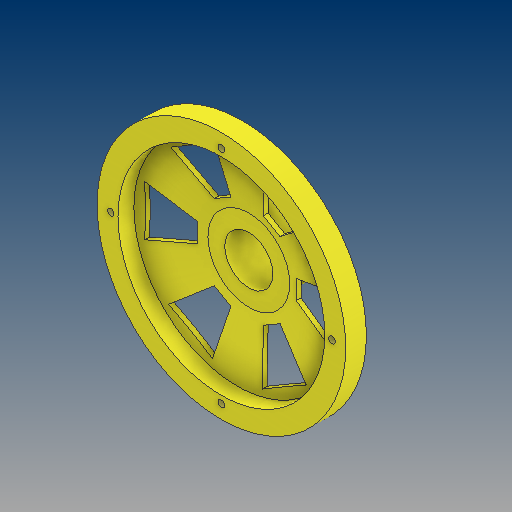
# Autodesk Inventor part: ring_1-sun_2
Saved by Autodesk Inventor 2021 (Build 250183000, 183)
## iProperties
Created: 2020-12-25
Part Number: ring_1-sun_2
Material: Generic
Document SubType Name: Modeling
Designer: Διογενης Τσιχλακης
Density: 1 g/cm^3
Appearance: Default
Mass: 1678.65 g
Surface Area: 4498.74 cm^2
Volume: 1678.65 cm^3
Sending System: Autodesk Inventor 2021
Preprocessor: unknown
Minimum Resolution: 0.01
Sent Units: Millimeter
Translation Standard: IGES 5.3
Model Creation Time: 2020-12-25
Title: sun_2_narrow
Author: Angelos
Autodesk Inventor part; units mm, degrees
ref_plane "YZ Plane" through (0, 0, 0) normal (1, 0, 0) x (0, 1, 0)
ref_plane "XZ Plane" through (0, 0, 0) normal (0, 1, 0) x (-1, 0, 0)
ref_plane "Work Plane1" through (-79.7284, -22.4294, -13.998) normal (0, 0, -1) x (-0.9355686, -0.3531449, 0)
sketch "Sketch5" plane through (-79.7284, -22.4294, -13.998) normal (0, 0, -1) x (-0.9355686, -0.3531449, 0)
  circle A0 centre (-82.5122, -7.1715) radius 70
  circle A1 centre (-82.5122, -7.1715) radius 50
  dimension "d4" = 100
  dimension "d30" = 140
  constraints: 2 centre point, 2 coincident
  measures "d4" diameter of A1
  measures "d30" diameter of A0
extrude "Extrusion2" add sketch "Sketch5" against normal blind 77
sketch "Sketch6" plane through (0, 0, 63.002) normal (0, 0, 1) x (1, 0, 0)
  circle A0 centre (0, 0) radius 85
  circle A1 centre (0, 0) radius 50
  dimension "d7" = 170
  dimension "d8" = 100
  constraints: 2 centre point, 2 coincident
  measures "d7" diameter of A0
  measures "d8" diameter of A1
extrude "Extrusion3" add sketch "Sketch6" along normal blind 10
sketch "Sketch7" plane through (0, 0, 0) normal (0, 1, 0) x (-1, 0, 0)
  line L0 (85, 73.002) -> (-85, 73.002) projected
  line L1 (-215, 97) -> (-85, 73.002)
  line L2 (85, 63.002) -> (-85, 63.002) projected
  line L3 (-85, 73.002) -> (-85, 63.002)
  line L4 (-215, 97) -> (-215, 87)
  line L5 (-215, 87) -> (-85, 63.002)
  line L6 (-230, 87) -> (-215, 87)
  line L7 (-215, 97) -> (-230, 97)
  line L8 (0, -19.4) -> (0, 116.4) projected
  line L9 (-258.5, 87) -> (-258.5, 97)
  line L10 (-258.5, 97) -> (-230, 97)
  line L11 (0, 62) -> (-85, 62)
  line L12 (-215, 87) -> (-258.5, 87)
  point P0 (0, 0)
  dimension "d32" = 10
  dimension "d59" = 258.5
  constraints: 20 end point, 4 perpendicular, 3 horizontal, 2 point on line, 1 vertical
  measures "d32" distance between parallel lines of L6 L7
  measures "d59" distance from line of L8 L9.end
revolve "Revolution1" add sketch "Sketch7" angle 360 about axis through (0, 0, -10) along (0, 0, 1) contours L3 L5 L4 L1 | L4 L6 L12 L9 L10 L7
sketch "Sketch9" plane through (0, 0, 0) normal (0, 0, 1) x (1, 0, 0)
  line L0 (194.9339, 0) -> (194.9339, -55)
  line L1 (194.9339, 0) -> (194.9339, 50)
  line L2 (102.2316, 0) -> (102.2316, 20)
  line L3 (102.2316, 0) -> (102.2316, -20)
  line L4 (102.2316, -20) -> (194.9339, -55)
  line L5 (102.2316, 20) -> (194.9339, 50)
  point P0 (0, 0)
  constraints: 12 end point, 4 vertical
extrude "Extrusion5" cut sketch "Sketch9" along normal through all
pattern_circular "Circular Pattern2" count 6 over 360 about axis through (0, 0, -10) along (0, 0, 1) of "Extrusion5"
sketch "Sketch11" plane through (0, 0, 97) normal (0, 0, 1) x (1, 0, 0)
  circle A0 centre (0, 0) radius 258.5
  circle A1 centre (0, 0) radius 215
  dimension "d58" = 517
  constraints: 2 centre point, 2 coincident
  measures "d58" diameter of A0
extrude "Extrusion9" add sketch "Sketch11" along normal blind 33.07
sketch "Sketch12" plane through (0, 0, 130.07) normal (0, 0, 1) x (1, 0, 0)
  circle A0 centre (0, 230) radius 7
  point P0 (0, 0)
  dimension "d41" = 14
  dimension "d42" = 230
  constraints: 1 centre point
  measures "d41" diameter of A0
  measures "d42" distance of A0.centre point (0, 0)
extrude "Extrusion10" cut sketch "Sketch12" against normal blind 25
pattern_circular "Circular Pattern4" count 4 over 360 about axis through (0, 0, -13.998) along (0, 0, 1) of "Extrusion10"
sketch "Sketch14" plane through (0, 0, 0) normal (1, 0, 0) x (0, 1, 0)
  line L0 (237, 105.07) -> (227, 105.07)
  line L1 (230, 119.807) -> (237, 123.07)
  line L2 (237, 123.07) -> (230, 123.07)
  line L3 (223, 105.07) -> (237, 105.07) projected
  line L4 (230, 123.07) -> (230, 119.807)
  point P0 (0, 0)
  constraints: 8 end point, 1 horizontal, 1 perpendicular, 1 other
thread "Thread5" size "M14x2" class "6H" standard "ANSI Metric M Profile" full length
thread "Thread6" size "M14x2" class "6H" standard "ANSI Metric M Profile" full length
thread "Thread7" size "M14x2" class "6H" standard "ANSI Metric M Profile" full length
thread "Thread8" size "M14x2" class "6H" standard "ANSI Metric M Profile" full length
revolve "Revolution4" cut sketch "Sketch14" angle 360 about axis through (0, 230, 123.07) along (0, 0, -1)
pattern_circular "Circular Pattern5" count 4 over 360 about axis through (0, 0, 97) along (0, 0, 1) of "Revolution4"
sketch "Sketch16" plane through (0, 0, -13.998) normal (0, 0, -1) x (-1, 0, 0)
  circle A0 centre (-59, 0) radius 6
  circle A1 centre (0, 0) radius 85 projected
  dimension "d77" = 59
  dimension "d78" = 12
  constraints: 1 centre point
  measures "d77" distance of A1.centre A0.centre
  measures "d78" diameter of A0
extrude "Extrusion12" cut sketch "Sketch16" against normal blind 10 contours A0
sketch "Sketch17" plane through (0, 0, 0) normal (0, 1, 0) x (-1, 0, 0)
  line L0 (-53, -3.998) -> (-65, -3.998) projected
  line L1 (-70, -13.998) -> (70, -13.998) projected
  line L2 (-65, -3.998) -> (-53, -3.998)
  line L3 (-65, -3.998) -> (-59, 2.002)
  line L4 (-65, -3.998) -> (-48.2122, -3.998) construction
  line L5 (-59, 2.002) -> (-53, -3.998)
  line L6 (-59, 2.002) -> (-59, -3.998)
  point P0 (0, 0)
  dimension "d82" = 45
  dimension "d83" = 45
  constraints: 10 end point, 1 collinear, 1 horizontal, 1 perpendicular, 1 point on line
  measures "d82" angle of L4 L3
  measures "d83" angle of L0 L5
revolve "Revolution5" cut sketch "Sketch17" angle 360 about axis through (59, 0, 2.002) along (0, 0, -1) contours L0 L3 L6
pattern_circular "Circular Pattern6" count 5 over 360 about axis through (0, 0, -10) along (0, 0, 1) of "Extrusion12", "Revolution5"
thread "Thread9" size "M12x1.75" class "6H" standard "ANSI Metric M Profile" full length
thread "Thread10" size "M12x1.75" class "6H" standard "ANSI Metric M Profile" full length
thread "Thread11" size "M12x1.75" class "6H" standard "ANSI Metric M Profile" full length
thread "Thread12" size "M12x1.75" class "6H" standard "ANSI Metric M Profile" full length
thread "Thread13" size "M12x1.75" class "6H" standard "ANSI Metric M Profile" full length
sketch "Sketch18" plane through (0, 0, 0) normal (0, 1, 0) x (-1, 0, 0)
  line L0 (223, 105.07) -> (237, 105.07) projected
  line L1 (237, 105.07) -> (230, 98.07)
  line L2 (237, 105.07) -> (246.2767, 105.07) construction
  line L3 (223, 105.07) -> (230, 98.07)
  line L4 (223, 105.07) -> (237.4265, 105.07) construction
  line L5 (230, 98.07) -> (230, 105.07)
  line L6 (230, 98.07) -> (237, 98.07) construction
  line L7 (237, 105.07) -> (230, 105.07)
  point P0 (0, 0)
  dimension "d98" = 135
  dimension "d99" = 45
  dimension "d100" = 90
  constraints: 14 end point, 3 horizontal, 1 collinear, 1 perpendicular, 1 point on line
  measures "d98" angle of L1 L2
  measures "d99" angle of L3 L4
  measures "d100" angle of L6 L5
revolve "Revolution6" cut sketch "Sketch18" angle 360 about axis through (-230, 0, 98.07) along (0, 0, 1) contours L0 L1 L5
pattern_circular "Circular Pattern7" count 4 over 360 about axis through (0, 0, -10) along (0, 0, 1) of "Revolution6"
body "Solid2"
